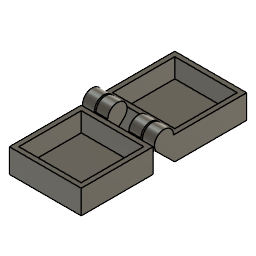
day-20-3d-printable-hinges (Autodesk Fusion 360 design; units mm, degrees)
part number: 2026-06-15-16-36-41-616
part number: 2026-06-15-16-39-09-046
part number: 2026-06-15-16-44-52-718
Autodesk Fusion 360 part; units mm, degrees
sketch "box width" plane through (0, 0, 0) normal (0, 0, 1) x (1, 0, 0) in component "box bottom"
  line L0 (0, 0) -> (30, 0)
  line L1 (30, 0) -> (30, 30)
  line L2 (30, 30) -> (0, 30)
  line L3 (0, 30) -> (0, 0)
  dimension "d3" = 30
  dimension "d4" = 30
  constraint horizontal L0
  constraint vertical L1
  constraint horizontal L2
  constraint vertical L3
  constraint coincident L0.start L3.end
  measures "d3" distance of L0.start L0.end
  measures "d4" distance of L0.start L2.end
extrude "Extrude1" add sketch "box width" along normal blind 10 makes body 1 in component "box bottom"
shell "Shell1" thickness 2 removed faces 1 at (10, 20, 10) on bodies 1 in component "box bottom"
sketch "box width (2)" plane through (0, 0, 0) normal (0, 0, 1) x (1, 0, 0) in component "box top"
  line L0 (0, 0) -> (30, 0)
  line L1 (30, 0) -> (30, 30)
  line L2 (30, 30) -> (0, 30)
  line L3 (0, 30) -> (0, 0)
  dimension "d3_1" = 30
  dimension "d4_1" = 30
  constraint horizontal L0
  constraint vertical L1
  constraint horizontal L2
  constraint vertical L3
  constraint coincident L0.start L3.end
  measures "d3_1" distance of L0.start L0.end
  measures "d4_1" distance of L0.start L2.end
extrude "Extrude1'" add sketch "box width (2)" along normal blind 10 separate body makes body 2 in component "box top"
shell "Shell1'" thickness 2 removed faces 1 at (10, 20, 10) on bodies 2 in component "box top"
sketch "side profile" plane through (0, 0, 0) normal (-1, 0, 0) x (0, -1, 0) in component "box bottom"
  line L0 (-30, 0) -> (0, 0)
  line L1 (0, 0) -> (0, 10)
  line L2 (0, 10) -> (-30, 10)
  line L3 (-30, 10) -> (-30, 0)
  line L4 (0, 10) -> (4.5, 10)
  circle A0 centre (4.5, 10) radius 4
  line L5 (0, 0) -> (7.2976, 7.1411)
  dimension "d16" = 4.5
  dimension "d17" = 8
  constraint coincident L1.end L2.start
  constraint perpendicular L1 L4
  constraint coincident L4.end A0.centre
  constraint coincident L0.end L1.start
  constraint coincident A0 L5.end
  constraint tangent A0 L5
  measures "d16" distance of L1.end L4.end
  measures "d17" diameter of A0
extrude "Extrude2" add sketch "side profile" against normal blind 5 separate body contours L1 L4 A0 L5 | A0 makes body 3 in component "box bottom"
sketch "Sketch3" plane through (5, 0, 0) normal (1, 0, 0) x (0, 1, 0) in component "box bottom"
  line L0 (0, 0) -> (0, 10)
  line L1 (0, 10) -> (-0.5, 10)
  arc A0 (-0.5, 10) -> (-7.2976, 7.1411) centre (-4.5, 10) ccw
  line L2 (-7.2976, 7.1411) -> (0, 0)
  arc A1 (-0.5, 10) -> (-7.2976, 7.1411) centre (-4.5, 10) ccw
  circle A2 centre (-4.5, 10) radius 2
  dimension "d20" = 4
  constraint concentric A0 A2
  measures "d20" diameter of A2
extrude "Extrude3" add sketch "Sketch3" along normal blind 3.8 draft -14 contours A2 bodies 3 in component "box bottom"
fillet "Fillet1" radius 1 1 edges at (8.8, -5.4813, 10.3806) on bodies 3 in component "box bottom"
sketch "hinge profile" plane through (25, 0, 0) normal (-1, 0, 0) x (0, -1, 0) in component "box top"
  circle A0 centre (4.5, 10) radius 2
  line L0 (9, 0) -> (9, 10)
  line L1 (9, 10) -> (8.5, 10)
  arc A1 (8.5, 10) -> (1.7024, 7.1411) centre (4.5, 10) ccw
  line L2 (1.7024, 7.1411) -> (9, 0)
  arc A2 (8.5, 10) -> (1.7024, 7.1411) centre (4.5, 10) ccw
  circle A3 centre (4.5, 10) radius 4
  line L3 (0, 10) -> (0.5, 10)
  line L4 (0, 0) -> (7.2976, 7.1411)
  line L5 (0, 0) -> (0, 10)
  constraint concentric A2 A3
  constraint coincident A1.end A3
  constraint coincident A1 L3.end
  constraint horizontal L3
  constraint coincident L4.start L5.start
  constraint coincident A3 L4.end
  constraint tangent A3 L4
extrude "Extrude2'" add sketch "hinge profile" along normal blind 5 from surface at 0.6 separate body contours A0 | A1 L2 A2 A3 L3 L4 L5 | L2 A3 L4 | A1 A2 A3 makes body 4 in component "box top"
combine "Combine1" operation cut target body 4 tool bodies 3 body 3 seen with x (-1, 0, 0) y (0, -1, 0) z (0, 0, 1) at (30, -9, 0) keep tools in component "box top"
move_face "OffsetFaces1" offset -0.4 3 faces at (21.2, -4.4436, 9.876) (21.8641, -5.6556, 9.6309) (23.8574, -3.4306, 8.6591) on bodies 4 in component "box top"
ref_plane "WorkPlane1" through (15, -24, 5) normal (1, 0, 0) x (0, 1, 0)
mirror "Mirror1" about plane through (15, -24, 5) normal (1, 0, 0) of bodies 3 makes body 5 in component "box bottom"
mirror "Mirror1'" about plane through (15, 15, 5) normal (-1, 0, 0) of bodies 4 makes body 6 in component "box top"
combine "Combine1'" operation add target body 1 tool bodies 5 3 in component "box bottom"
component "box bottom" placed x (1, 0, 0) y (0, 1, 0) z (0, 0, 1) at (0, 0, 0)
component "box top" placed x (-1, 0, 0) y (0, -1, 0) z (0, 0, 1) at (30, -9, 0)
equation "BoxWidth = 30 mm"
equation "BoxHeight = 20 mm"
equation "d3 = BoxWidth"
equation "d4 = BoxWidth"
equation "d5 = BoxHeight / 2"
equation "WallThickness = 2 mm"
equation "d3_1 = BoxWidth"
equation "d4_1 = BoxWidth"
equation "d5_1 = BoxHeight / 2"
equation "WallThickness_1 = 2 mm"
